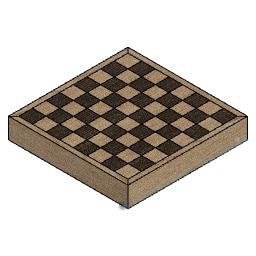
Chessboard (Autodesk Fusion 360 design; units mm, degrees)
Autodesk Fusion 360 part; units mm, degrees
note: some values were not read from the file. Chosen so that the rebuilt part matches the saved one: which bodies a step acts on.
sketch "Sketch1" plane through (0, 0, 0) normal (0, 0, 1) x (1, 0, 0)
  line L0 (0, 0) -> (-406.4051, 0)
  line L1 (-406.4051, 0) -> (-406.4051, 406.4)
  line L2 (-406.4051, 406.4) -> (0, 406.4)
  line L3 (0, 406.4) -> (0, 0)
  dimension "d1" = 406.4
  constraint horizontal L0
  constraint vertical L1
  constraint horizontal L2
  constraint vertical L3
  constraint coincident L0.start L3.end
  measures "d1" distance of L0.start L2.end
sketch "Sketch2" plane through (0, 0, 0) normal (0, 0, 1) x (1, 0, 0)
  line L0 (-406.4, 406.4) -> (0, 406.4)
  line L1 (0, 406.4) -> (0, 355.6)
  line L2 (0, 355.6) -> (-406.4, 355.6)
  line L3 (-406.4, 355.6) -> (-406.4, 406.4)
  line L4 (-406.4, 355.6) -> (0, 355.6)
  line L5 (0, 355.6) -> (0, 304.8)
  line L6 (0, 304.8) -> (-406.4, 304.8)
  line L7 (-406.4, 304.8) -> (-406.4, 355.6)
  line L8 (-406.4, 304.8) -> (0, 304.8)
  line L9 (0, 304.8) -> (0, 254)
  line L10 (0, 254) -> (-406.4, 254)
  line L11 (-406.4, 254) -> (-406.4, 304.8)
  line L12 (-406.4, 254) -> (0, 254)
  line L13 (0, 254) -> (0, 203.2)
  line L14 (0, 203.2) -> (-406.4, 203.2)
  line L15 (-406.4, 203.2) -> (-406.4, 254)
  line L16 (-406.4, 203.2) -> (0, 203.2)
  line L17 (0, 203.2) -> (0, 152.4)
  line L18 (0, 152.4) -> (-406.4, 152.4)
  line L19 (-406.4, 152.4) -> (-406.4, 203.2)
  line L20 (-406.4, 152.4) -> (0, 152.4)
  line L21 (0, 152.4) -> (0, 101.6)
  line L22 (0, 101.6) -> (-406.4, 101.6)
  line L23 (-406.4, 101.6) -> (-406.4, 152.4)
  line L24 (-406.4, 101.6) -> (0, 101.6)
  line L25 (0, 101.6) -> (0, 50.8)
  line L26 (0, 50.8) -> (-406.4, 50.8)
  line L27 (-406.4, 50.8) -> (-406.4, 101.6)
  line L28 (-406.4, 50.8) -> (0, 50.8)
  line L29 (0, 50.8) -> (0, 0)
  line L30 (0, 0) -> (-406.4, 0)
  line L31 (-406.4, 0) -> (-406.4, 50.8)
  line L32 (-406.4, 406.4) -> (-355.6, 406.4)
  line L33 (-355.6, 406.4) -> (-355.6, 0)
  line L34 (-355.6, 0) -> (-406.4, 0)
  line L35 (-406.4, 0) -> (-406.4, 406.4)
  line L36 (-355.6, 0) -> (-304.8, 0)
  line L37 (-304.8, 0) -> (-304.8, 406.4)
  line L38 (-304.8, 406.4) -> (-355.6, 406.4)
  line L39 (-355.6, 406.4) -> (-355.6, 0)
  line L40 (-304.8, 406.4) -> (-254, 406.4)
  line L41 (-254, 406.4) -> (-254, 0)
  line L42 (-254, 0) -> (-304.8, 0)
  line L43 (-304.8, 0) -> (-304.8, 406.4)
  line L44 (-254, 0) -> (-203.2, 0)
  line L45 (-203.2, 0) -> (-203.2, 406.4)
  line L46 (-203.2, 406.4) -> (-254, 406.4)
  line L47 (-254, 406.4) -> (-254, 0)
  line L48 (-203.2, 406.4) -> (-152.4, 406.4)
  line L49 (-152.4, 406.4) -> (-152.4, 0)
  line L50 (-152.4, 0) -> (-203.2, 0)
  line L51 (-203.2, 0) -> (-203.2, 406.4)
  line L52 (-152.4, 0) -> (-101.6, 0)
  line L53 (-101.6, 0) -> (-101.6, 406.4)
  line L54 (-101.6, 406.4) -> (-152.4, 406.4)
  line L55 (-152.4, 406.4) -> (-152.4, 0)
  line L56 (-101.6, 406.4) -> (-50.8, 406.4)
  line L57 (-50.8, 406.4) -> (-50.8, 0)
  line L58 (-50.8, 0) -> (-101.6, 0)
  line L59 (-101.6, 0) -> (-101.6, 406.4)
  constraint horizontal L0
  constraint vertical L1
  constraint horizontal L2
  constraint vertical L3
  constraint horizontal L4
  constraint vertical L5
  constraint horizontal L6
  constraint vertical L7
  constraint horizontal L8
  constraint vertical L9
  constraint horizontal L10
  constraint vertical L11
  constraint horizontal L12
  constraint vertical L13
  constraint horizontal L14
  constraint vertical L15
  constraint horizontal L16
  constraint vertical L17
  constraint horizontal L18
  constraint vertical L19
  constraint horizontal L20
  constraint vertical L21
  constraint horizontal L22
  constraint vertical L23
  constraint horizontal L24
  constraint vertical L25
  constraint horizontal L26
  constraint vertical L27
  constraint horizontal L28
  constraint vertical L29
  constraint horizontal L30
  constraint vertical L31
  constraint coincident L29.end L30.start
  constraint horizontal L32
  constraint vertical L33
  constraint horizontal L34
  constraint vertical L35
  constraint horizontal L36
  constraint vertical L37
  constraint horizontal L38
  constraint vertical L39
  constraint coincident L0 L37.end
  constraint horizontal L40
  constraint vertical L41
  constraint horizontal L42
  constraint vertical L43
  constraint coincident L30 L41.end
  constraint horizontal L44
  constraint vertical L45
  constraint horizontal L46
  constraint vertical L47
  constraint midpoint L0 L45.end
  constraint horizontal L48
  constraint vertical L49
  constraint horizontal L50
  constraint vertical L51
  constraint horizontal L52
  constraint vertical L53
  constraint horizontal L54
  constraint vertical L55
  constraint coincident L0 L53.end
  constraint horizontal L56
  constraint vertical L57
  constraint horizontal L58
  constraint vertical L59
  constraint coincident L30 L57.end
extrude "Extrude3" add sketch "Sketch1" along normal blind 6.35 makes body 1
sketch "Sketch4" plane through (0, 0, 6.35) normal (0, 0, 1) x (-1, 0, 0)
  line L0 (0, -406.4) -> (406.4051, -406.4)
  line L1 (406.4051, -406.4) -> (406.4051, 0)
  line L2 (406.4051, 0) -> (0, 0)
  line L3 (0, 0) -> (0, -406.4)
  line L4 (406.4051, -355.6) -> (0, -355.6)
  line L5 (406.4051, -304.8) -> (0, -304.8)
  line L6 (0, -254) -> (406.4051, -254)
  line L7 (406.4051, -203.2) -> (0, -203.2)
  line L8 (0, -152.4) -> (406.4051, -152.4)
  line L9 (406.4051, -101.6) -> (0, -101.6)
  line L10 (0, -50.8) -> (406.4051, -50.8)
  line L11 (355.6051, -406.4) -> (355.6051, 0)
  line L12 (304.8, 0) -> (304.8, -406.4)
  line L13 (254, 0) -> (254, -406.4)
  line L14 (203.2026, 0) -> (203.2026, -406.4)
  line L15 (152.4, 0) -> (152.4, -406.4)
  line L16 (101.6, 0) -> (101.6, -406.4)
  line L17 (50.8, 0) -> (50.8, -406.4)
  line L18 (406.4051, -406.4) -> (0, -406.4)
  line L19 (0, -406.4) -> (0, 0)
  line L20 (0, 0) -> (406.4051, 0)
  line L21 (406.4051, 0) -> (406.4051, -406.4)
  dimension "d8" = 50.8
  dimension "d9" = 50.8
  constraint coincident L1 L4.start
  constraint coincident L3 L4.end
  constraint perpendicular L3 L4
  constraint coincident L1 L5.start
  constraint coincident L3 L5.end
  constraint perpendicular L3 L5
  constraint coincident L3 L6.start
  constraint coincident L1 L6.end
  constraint perpendicular L1 L6
  constraint midpoint L1 L7.start
  constraint midpoint L3 L7.end
  constraint coincident L3 L8.start
  constraint coincident L1 L8.end
  constraint perpendicular L1 L8
  constraint coincident L1 L9.start
  constraint coincident L3 L9.end
  constraint perpendicular L3 L9
  constraint coincident L1 L10.end
  constraint perpendicular L1 L10
  constraint coincident L2 L11.end
  constraint perpendicular L2 L11
  constraint coincident L2 L12.start
  constraint coincident L0 L12.end
  constraint perpendicular L0 L12
  constraint coincident L2 L13.start
  constraint coincident L0 L13.end
  constraint perpendicular L0 L13
  constraint midpoint L2 L14.start
  constraint midpoint L0 L14.end
  constraint coincident L2 L15.start
  constraint coincident L0 L15.end
  constraint perpendicular L0 L15
  constraint coincident L2 L16.start
  constraint coincident L0 L16.end
  constraint perpendicular L0 L16
  constraint coincident L2 L17.start
  constraint coincident L0 L17.end
  constraint perpendicular L0 L17
  constraint coincident L0.end L1.start
  constraint coincident L0.start L3.end
  constraint coincident L2.end L3.start
  constraint coincident L1.end L2.start
  measures "d8" distance of L9.end L10.start
  measures "d9" distance of L0.end L11.start
split "Split1" by curves path "Sketch4" along L7 L6 L5 L4 L8 L9 L10 bodies 1 makes body 2 at (-135.4684, 118.5333, 0) makes body 3 at (-135.4684, 372.5333, 0) makes body 4 at (-135.4684, 67.7333, 0) makes body 5 at (-135.4684, 220.1333, 0) makes body 6 at (-135.4684, 321.7333, 0) makes body 7 at (-135.4684, 169.3333, 0) makes body 8 at (-135.4684, 270.9333, 0)
sketch "Sketch5" plane through (0, 0, 6.35) normal (0, 0, 1) x (-1, 0, 0)
  line L0 (406.4051, -355.6) -> (0, -355.6)
  line L1 (0, -355.6) -> (0, -406.4)
  line L2 (0, -406.4) -> (406.4051, -406.4)
  line L3 (406.4051, -406.4) -> (406.4051, -355.6)
  line L4 (406.4051, -406.4) -> (355.6, -406.4)
  line L5 (355.6, -406.4) -> (355.6, 0)
  constraint coincident L2.end L3.start
  constraint coincident L2 L4.end
  constraint perpendicular L3 L4
  constraint perpendicular L0 L5
split "Split2" by curves path "Sketch5" along L4 L5 bodies 8 6 5 7 2 4 1 3 makes body 16 at (-237.0667, 389.4667, 0) makes body 15 at (-237.0667, 33.8667, 0) makes body 14 at (-118.5333, 67.7333, 0) makes body 13 at (-118.5333, 118.5333, 0) makes body 12 at (-237.0667, 186.2667, 0) makes body 11 at (-237.0667, 220.1333, 0) makes body 10 at (-118.5333, 321.7333, 0) makes body 9 at (-237.0667, 287.8667, 0)
sketch "Sketch6" plane through (0, 0, 6.35) normal (0, 0, 1) x (-1, 0, 0)
  line L0 (355.6, -406.4) -> (355.6, -355.6)
  line L1 (355.6, -355.6) -> (0, -355.6)
  line L2 (0, -355.6) -> (0, -406.4)
  line L3 (0, -406.4) -> (355.6, -406.4)
  line L4 (304.8, 0) -> (304.8, -406.4)
  line L5 (254, -406.4) -> (254, 0)
  line L6 (203.2, 0) -> (203.2, -406.4)
  line L7 (152.4, -406.4) -> (152.4, 0)
  line L8 (101.6, 0) -> (101.6, -406.4)
  line L9 (50.8, -406.4) -> (50.8, 0)
  constraint coincident L3 L4.end
  constraint coincident L3 L5.start
  constraint coincident L3 L6.end
  constraint perpendicular L3 L6
  constraint coincident L3 L7.start
  constraint coincident L3 L8.end
  constraint perpendicular L3 L8
  constraint coincident L3 L9.start
split "Split3" by curves path "Sketch6" along L4 L5 L6 L7 L8 L9 bodies 10 9 11 12 13 14 15 16 makes body 59 at (-16.9333, 372.5333, 0) makes body 60 at (-118.5333, 372.5333, 0) makes body 61 at (-220.1333, 372.5333, 0) makes body 62 at (-67.7333, 372.5333, 0) makes body 63 at (-169.3333, 372.5333, 0) makes body 64 at (-270.9333, 372.5333, 0) makes body 53 at (-16.9333, 33.8667, 0) makes body 54 at (-135.4667, 16.9333, 0) makes body 55 at (-237.0667, 16.9333, 0) makes body 56 at (-67.7333, 16.9333, 0) makes body 57 at (-169.3333, 16.9333, 0) makes body 58 at (-270.9333, 16.9333, 0) makes body 47 at (-33.8667, 84.6667, 0) makes body 48 at (-135.4667, 84.6667, 0) makes body 49 at (-237.0667, 84.6667, 0) makes body 50 at (-84.6667, 84.6667, 0) makes body 51 at (-186.2667, 84.6667, 0) makes body 52 at (-287.8667, 84.6667, 0) makes body 41 at (-16.9333, 118.5333, 0) makes body 42 at (-118.5333, 118.5333, 0) makes body 43 at (-220.1333, 118.5333, 0) makes body 44 at (-67.7333, 118.5333, 0) makes body 45 at (-169.3333, 118.5333, 0) makes body 46 at (-270.9333, 118.5333, 0) makes body 35 at (-33.8667, 186.2667, 0) makes body 36 at (-135.4667, 186.2667, 0) makes body 37 at (-237.0667, 186.2667, 0) makes body 38 at (-84.6667, 186.2667, 0) makes body 39 at (-186.2667, 186.2667, 0) makes body 40 at (-287.8667, 186.2667, 0) makes body 29 at (-16.9333, 220.1333, 0) makes body 30 at (-118.5333, 220.1333, 0) makes body 31 at (-220.1333, 220.1333, 0) makes body 32 at (-67.7333, 220.1333, 0) makes body 33 at (-169.3333, 220.1333, 0) makes body 34 at (-270.9333, 220.1333, 0) makes body 23 at (-33.8667, 287.8667, 0) makes body 24 at (-135.4667, 287.8667, 0) makes body 25 at (-237.0667, 287.8667, 0) makes body 26 at (-84.6667, 287.8667, 0) makes body 27 at (-186.2667, 287.8667, 0) makes body 28 at (-287.8667, 287.8667, 0) makes body 17 at (-16.9333, 321.7333, 0) makes body 18 at (-118.5333, 321.7333, 0) makes body 19 at (-220.1333, 321.7333, 0) makes body 20 at (-67.7333, 321.7333, 0) makes body 21 at (-169.3333, 321.7333, 0) makes body 22 at (-270.9333, 321.7333, 0)
move_body "Move1" bodies 1 30 18 4 45 42 39 52 53 63 64 19 24 21 41 38 35 20 59 47 48 33 57 34 50 54 43 23 22 56 36 62 32 16 31 15 46 17 49 29 25 44 40 26 51 60 8 7 27 6 9 28 10 11 61 2 37 14 12 58 13 55 3 to x (1, 0, 0) y (0, 1, 0) z (0, 0, 1) at (0, 0, 76.2)
sketch "Sketch7" plane through (0, 0, 0) normal (0, 0, 1) x (1, 0, 0)
  line L0 (0, 0) -> (0, -19.05)
  line L1 (0, 406.4) -> (0, 425.45)
  line L2 (0, 425.45) -> (19.0421, 425.45)
  line L3 (19.0421, 425.45) -> (19.0421, -19.05)
  line L4 (19.0421, -19.05) -> (0, -19.05)
  line L5 (0, -19.05) -> (0, 425.45)
  dimension "d10" = 19.05
  dimension "d11" = 19.05
  constraint coincident L0.start origin
  constraint vertical L0
  constraint vertical L1
  constraint horizontal L2
  constraint vertical L3
  constraint horizontal L4
  constraint vertical L5
  measures "d10" distance of L0.start L0.end
  measures "d11" distance of L1.start L1.end
sketch "Sketch8" plane through (0, 0, 0) normal (0, 0, 1) x (1, 0, 0)
  line L0 (0, 406.4) -> (19.0813, 425.4798)
  line L1 (0, 0) -> (19.05, -19.05)
  line L2 (0, 406.4) -> (0, 0)
  line L3 (0, 406.4) -> (0, 0)
  line L4 (19.05, -19.05) -> (19.0813, 425.4798)
  line L5 (0, 406.4) -> (19.0813, 425.4798)
  constraint coincident L1.start L2.end
  constraint vertical L2
  constraint parallel L0 L5
extrude "Extrude4" add sketch "Sketch8" along normal blind 76.2 separate body makes body 65
move_body "Move2" bodies 64 30 18 4 45 42 39 52 53 63 1 19 24 21 41 38 35 20 59 47 48 33 57 34 50 54 43 23 22 56 36 62 32 16 31 15 46 17 49 29 25 44 40 26 51 60 8 7 27 6 9 28 10 11 61 2 37 14 12 58 13 55 3 to x (1, 0, 0) y (0, 1, 0) z (0, 0, 1) at (0, 0, -6.35)
move_body "Move3" bodies 5 to x (1, 0, 0) y (0, 1, 0) z (0, 0, 1) at (0, 0, 69.85)
sketch "Sketch9" plane through (0, 0, 0) normal (0, 0, 1) x (1, 0, 0)
copy_body "CopyPasteBodies1" bodies 65 makes body 66
move_body "Move4" bodies 66 to x (0, -1, 0) y (1, 0, 0) z (0, 0, 1) at (-406.4, 0, 0)
copy_body "CopyPasteBodies3" bodies 65 makes body 67
move_body "Move6" bodies 67 to x (-1, 0, 0) y (0, 1, 0) z (0, 0, -1) at (0, 0, 0)
move_body "Move7" bodies 67 to x (0, -1, 0) y (1, 0, 0) z (0, 0, 1) at (-406.4313, 406.3687, 0)
copy_body "CopyPasteBodies4" bodies 65 makes body 68
move_body "Move8" bodies 68 to x (-1, 0, 0) y (0, -1, 0) z (0, 0, 1) at (-406.4, 406.4, 0)
move_body "Move9" bodies 67 to x (1, 0, 0) y (0, 1, 0) z (0, 0, 1) at (0, 0, 76.2)
equation "d6 = ( 1 / 4 ) * 1 in"
